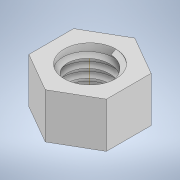
# Autodesk Inventor part: boltExample
Saved by Autodesk Inventor 2021.1 (Build 251245000, 245)
## iProperties
Created: 2020-06-15
Part Number: boltExample
Material: Generic
Document SubType Name: Modeling
Designer: robst
Density: 1 g/cm^3
Appearance: Default
Author: robst
Autodesk Inventor part; units mm, degrees
ref_plane "YZ Plane" through (0, 0, 0) normal (1, 0, 0) x (0, 1, 0)
ref_plane "XZ Plane" through (0, 0, 0) normal (0, 1, 0) x (-1, 0, 0)
ref_plane "XY Plane" through (0, 0, 0) normal (0, 0, 1) x (1, 0, 0)
sketch "Sketch1" plane through (0, 0, 0) normal (0, 1, 0) x (-1, 0, 0)
  line L0 (-7.1438, -4.1244) -> (-7.1438, 4.1244)
  line L1 (-7.1438, 4.1244) -> (0, 8.2489)
  line L2 (0, 8.2489) -> (7.1438, 4.1244)
  line L3 (7.1438, 4.1244) -> (7.1437, -4.1244)
  line L4 (7.1437, -4.1244) -> (0, -8.2489)
  line L5 (0, -8.2489) -> (-7.1438, -4.1244)
  point P0 (0, 0)
  point P1 (0, 0)
  dimension "d0" = 14.2875
  constraints: 12 end point, 1 coincident, 1 vertical, 13 other
  measures "d0" distance between parallel lines of L0 L3
extrude "Extrusion1" add sketch "Sketch1" against normal blind 8.3344
sketch "Sketch2" plane through (0, 0, 0) normal (0, 1, 0) x (1, 0, 0)
  circle A0 centre (0, 0) radius 4.7625
  dimension "d3" = 9.525
  constraints: 1 centre point, 1 coincident
  measures "d3" diameter of A0
extrude "Extrusion2" cut sketch "Sketch2" against normal through all
sketch "Sketch3" plane through (0, 0, 0) normal (1, 0, 0) x (0, 1, 0)
  line L0 (0, -4.7625) -> (-8.3344, -4.7625) projected
  line L1 (0, 4.7625) -> (0, -4.7625) projected
  line L2 (-10.188, 0) -> (2.7876, 0) projected
  line L3 (0, -4.7625) -> (-0.4986, -3.8989)
  line L4 (-0.4986, -3.8989) -> (-0.9972, -4.7625)
  point P0 (0, 0)
  dimension "d18" = 60
  dimension "d19" = 3.8989
  dimension "d20" = 30
  constraints: 4 end point, 1 equal length, 1 point on line
  measures "d18" angle of L4 L3
  measures "d19" distance from line of L3.end L2
  measures "d20" angle of L3 L1
coil "Coil2" sketch "Sketch3" operation add axis through (0, -10, 0) along (0, -1, 0) pitch 1.5875 turns 4.626 hand right
body "Solid1"
